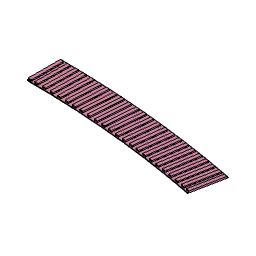
0_15m_Joch_Gebogen_Schablone (Autodesk Fusion 360 design; units mm, degrees)
Autodesk Fusion 360 part; units mm, degrees
sketch "Skizze4" plane through (0, 0, 0) normal (0, 0, 1) x (1, 0, 0)
  line L0 (0, 0) -> (0, -1665.39) construction
  circle A0 centre (0, -1665.39) radius 1665.39 construction
  line L1 (9.1953, 13.0775) -> (9.1001, -0.0222)
  line L2 (9.1001, -0.0222) -> (15.0999, -0.0658)
  line L3 (15.0999, -0.0658) -> (15.1951, 13.0339)
  line L4 (15.1951, 13.0339) -> (9.1953, 13.0775)
  line L5 (-3, 13.1) -> (3, 13.1)
  line L6 (3, 13.1) -> (3, 0)
  line L7 (3, 0) -> (-3, 0)
  line L8 (-3, 0) -> (-3, 13.1)
  line L9 (12.1952, 13.0557) -> (12.1, -0.044) construction
  line L10 (23.708, 12.9352) -> (23.4995, -0.1631)
  line L11 (29.4988, -0.2586) -> (29.7072, 12.8398)
  line L12 (26.7076, 12.8875) -> (26.4992, -0.2108) construction
  line L13 (29.7072, 12.8398) -> (23.708, 12.9352)
  line L14 (23.4995, -0.1631) -> (29.4988, -0.2586)
  line L15 (38.219, 12.6675) -> (37.8973, -0.4285)
  line L16 (58.7237, 12.0751) -> (52.7271, 12.2743)
  line L17 (52.2921, -0.8185) -> (58.2888, -1.0177)
  line L18 (52.7271, 12.2743) -> (52.2921, -0.8185)
  line L19 (58.2888, -1.0177) -> (58.7237, 12.0751)
  line L20 (55.7254, 12.1747) -> (55.2905, -0.9181) construction
  line L21 (41.218, 12.5938) -> (40.8964, -0.5022) construction
  line L22 (37.8973, -0.4285) -> (43.8954, -0.5759)
  line L23 (43.8954, -0.5759) -> (44.2171, 12.5202)
  line L24 (44.2171, 12.5202) -> (38.219, 12.6675)
  line L25 (115.808, -4.0287) -> (116.6954, 9.0412)
  line L26 (101.4385, -3.0895) -> (102.2129, 9.9876)
  line L27 (81.7303, 11.1117) -> (81.0691, -1.9716)
  line L28 (102.2129, 9.9876) -> (96.2234, 10.3423)
  line L29 (67.2312, 11.7557) -> (66.6831, -1.3328)
  line L30 (109.8218, -3.6223) -> (115.808, -4.0287)
  line L31 (87.7227, 10.8088) -> (81.7303, 11.1117)
  line L32 (66.6831, -1.3328) -> (72.6779, -1.5839)
  line L33 (70.2286, 11.6302) -> (69.6805, -1.4584) construction
  line L34 (113.7023, 9.2444) -> (112.8149, -3.8255) construction
  line L35 (81.0691, -1.9716) -> (87.0614, -2.2745)
  line L36 (72.6779, -1.5839) -> (73.226, 11.5046)
  line L37 (84.7265, 10.9602) -> (84.0653, -2.1231) construction
  line L38 (99.2181, 10.165) -> (98.4438, -2.9121) construction
  line L39 (96.2234, 10.3423) -> (95.449, -2.7348)
  line L40 (110.7092, 9.4477) -> (109.8218, -3.6223)
  line L41 (95.449, -2.7348) -> (101.4385, -3.0895)
  line L42 (116.6954, 9.0412) -> (110.7092, 9.4477)
  line L43 (73.226, 11.5046) -> (67.2312, 11.7557)
  line L44 (87.0614, -2.2745) -> (87.7227, 10.8088)
  line L45 (197.4125, 1.4531) -> (195.8485, -11.5532)
  line L46 (139.6549, 7.2828) -> (138.5417, -5.7698)
  line L47 (154.1127, 6.0127) -> (152.8866, -7.0298)
  line L48 (214.793, -0.7) -> (213.1166, -13.6923) construction
  line L49 (173.1887, -9.027) -> (174.5275, 4.0044)
  line L50 (171.5432, 4.3111) -> (170.2044, -8.7204) construction
  line L51 (138.5417, -5.7698) -> (144.52, -6.2797)
  line L52 (152.8866, -7.0298) -> (158.8603, -7.5914)
  line L53 (200.391, 1.095) -> (198.8271, -11.9113) construction
  line L54 (145.6332, 6.7729) -> (139.6549, 7.2828)
  line L55 (211.8177, -0.3161) -> (210.1413, -13.3084)
  line L56 (224.4184, -15.1872) -> (230.3622, -16.0064)
  line L57 (232.1508, -3.0291) -> (226.207, -2.2099)
  line L58 (125.1868, 8.4278) -> (124.1864, -4.634)
  line L59 (182.9926, 3.0978) -> (181.5411, -9.9216)
  line L60 (167.2201, -8.4137) -> (173.1887, -9.027)
  line L61 (217.7683, -1.084) -> (211.8177, -0.3161)
  line L62 (210.1413, -13.3084) -> (216.092, -14.0762)
  line L63 (229.1789, -2.6195) -> (227.3903, -15.5968) construction
  line L64 (185.9741, 2.7654) -> (184.5226, -10.254) construction
  line L65 (131.1692, 7.9696) -> (125.1868, 8.4278)
  line L66 (130.1688, -5.0922) -> (131.1692, 7.9696)
  line L67 (201.8056, -12.2695) -> (203.3696, 0.7368)
  line L68 (160.0864, 5.4511) -> (154.1127, 6.0127)
  line L69 (158.8603, -7.5914) -> (160.0864, 5.4511)
  line L70 (230.3622, -16.0064) -> (232.1508, -3.0291)
  line L71 (168.5589, 4.6177) -> (167.2201, -8.4137)
  line L72 (157.0995, 5.7319) -> (155.8734, -7.3106) construction
  line L73 (188.9556, 2.433) -> (182.9926, 3.0978)
  line L74 (142.6441, 7.0278) -> (141.5308, -6.0248) construction
  line L75 (187.5041, -10.5864) -> (188.9556, 2.433)
  line L76 (128.178, 8.1987) -> (127.1776, -4.8631) construction
  line L77 (203.3696, 0.7368) -> (197.4125, 1.4531)
  line L78 (181.5411, -9.9216) -> (187.5041, -10.5864)
  line L79 (174.5275, 4.0044) -> (168.5589, 4.6177)
  line L80 (195.8485, -11.5532) -> (201.8056, -12.2695)
  line L81 (226.207, -2.2099) -> (224.4184, -15.1872)
  line L82 (144.52, -6.2797) -> (145.6332, 6.7729)
  line L83 (216.092, -14.0762) -> (217.7683, -1.084)
  line L84 (124.1864, -4.634) -> (130.1688, -5.0922)
  line L85 (0, 13.1) -> (0, 0) construction
  line L86 (243.5477, -4.6633) -> (241.6469, -17.6247) construction
  line L87 (275.1899, -9.6098) -> (269.2693, -8.6366)
  line L88 (287.2601, -24.9588) -> (281.3482, -23.9345)
  line L89 (286.5405, -11.539) -> (284.3042, -24.4467) construction
  line L90 (269.2693, -8.6366) -> (267.1446, -21.5632)
  line L91 (246.516, -5.0986) -> (240.5795, -4.228)
  line L92 (281.3482, -23.9345) -> (283.5846, -11.0268)
  line L93 (244.6152, -18.06) -> (246.516, -5.0986)
  line L94 (252.9211, -19.3147) -> (258.8499, -20.2366)
  line L95 (289.4965, -12.0511) -> (287.2601, -24.9588)
  line L96 (240.5795, -4.228) -> (238.6787, -17.1894)
  line L97 (273.0652, -22.5363) -> (275.1899, -9.6098)
  line L98 (258.8499, -20.2366) -> (260.8627, -7.2922)
  line L99 (238.6787, -17.1894) -> (244.6152, -18.06)
  line L100 (254.9339, -6.3703) -> (252.9211, -19.3147)
  line L101 (283.5846, -11.0268) -> (289.4965, -12.0511)
  line L102 (260.8627, -7.2922) -> (254.9339, -6.3703)
  line L103 (272.2296, -9.1232) -> (270.1049, -22.0497) construction
  line L104 (257.8983, -6.8312) -> (255.8855, -19.7757) construction
  line L105 (267.1446, -21.5632) -> (273.0652, -22.5363)
  line L106 (315.0971, -16.7413) -> (312.6378, -29.6084) construction
  line L107 (318.0437, -17.3045) -> (312.1504, -16.1781)
  line L108 (321.6701, -31.3578) -> (327.555, -32.5273)
  line L109 (324.2235, -18.5091) -> (321.6701, -31.3578)
  line L110 (315.5845, -30.1716) -> (318.0437, -17.3045)
  line L111 (312.1504, -16.1781) -> (309.6912, -29.0452)
  line L112 (303.7815, -14.6161) -> (297.8786, -13.5407)
  line L113 (297.8786, -13.5407) -> (295.5307, -26.4286)
  line L114 (295.5307, -26.4286) -> (301.4336, -27.504)
  line L115 (300.83, -14.0784) -> (298.4822, -26.9663) construction
  line L116 (327.166, -19.0938) -> (324.6125, -31.9426) construction
  line L117 (301.4336, -27.504) -> (303.7815, -14.6161)
  line L118 (330.1084, -19.6786) -> (324.2235, -18.5091)
  line L119 (327.555, -32.5273) -> (330.1084, -19.6786)
  line L120 (309.6912, -29.0452) -> (315.5845, -30.1716)
  point P0 (12.1, -0.044)
  point P1 (26.4992, -0.2108)
  point P2 (55.2905, -0.9181)
  point P3 (40.8964, -0.5022)
  point P4 (112.8149, -3.8255)
  point P5 (98.4438, -2.9121)
  point P6 (84.0653, -2.1231)
  point P7 (69.6805, -1.4584)
  point P8 (170.2044, -8.7204)
  point P9 (155.8734, -7.3106)
  point P10 (198.8271, -11.9113)
  point P11 (184.5226, -10.254)
  point P12 (213.1166, -13.6923)
  point P13 (227.3903, -15.5968)
  point P14 (141.5308, -6.0248)
  point P15 (127.1776, -4.8631)
  point P16 (255.8855, -19.7757)
  point P17 (241.6469, -17.6247)
  point P18 (284.3042, -24.4467)
  point P19 (270.1049, -22.0497)
  point P20 (312.6378, -29.6084)
  point P21 (324.6125, -31.9426)
  point P22 (298.4822, -26.9663)
  dimension "d197" = 1665.39
  dimension "d198" = 6
  dimension "d199" = 13.1
  dimension "d200" = 6
  dimension "d201" = 13.1
  dimension "d202" = 6
  dimension "d203" = 13.1
  dimension "d204" = 6
  dimension "d205" = 13.1
  dimension "d206" = 6
  dimension "d207" = 13.1
  dimension "d208" = 6
  dimension "d209" = 13.1
  dimension "d210" = 6
  dimension "d211" = 13.1
  dimension "d212" = 6
  dimension "d213" = 13.1
  dimension "d214" = 6
  dimension "d215" = 13.1
  dimension "d216" = 6
  dimension "d217" = 13.1
  dimension "d218" = 6
  dimension "d219" = 13.1
  dimension "d220" = 6
  dimension "d221" = 13.1
  dimension "d222" = 6
  dimension "d223" = 13.1
  dimension "d224" = 6
  dimension "d225" = 13.1
  dimension "d226" = 6
  dimension "d227" = 13.1
  dimension "d228" = 6
  dimension "d229" = 13.1
  dimension "d230" = 6
  dimension "d231" = 13.1
  dimension "d232" = 12.1
  dimension "d233" = 14.4
  dimension "d234" = 14.4
  dimension "d235" = 14.4
  dimension "d236" = 14.4
  dimension "d237" = 14.4
  dimension "d238" = 14.4
  dimension "d239" = 14.4
  dimension "d240" = 6
  dimension "d241" = 13.1
  dimension "d242" = 6
  dimension "d243" = 13.1
  dimension "d244" = 6
  dimension "d245" = 13.1
  dimension "d246" = 6
  dimension "d247" = 13.1
  dimension "d248" = 6
  dimension "d249" = 13.1
  dimension "d250" = 6
  dimension "d251" = 13.1
  dimension "d252" = 6
  dimension "d253" = 13.1
  dimension "d254" = 14.4
  dimension "d255" = 14.4
  dimension "d256" = 14.4
  dimension "d257" = 14.4
  dimension "d258" = 14.4
  dimension "d259" = 14.4
  dimension "d260" = 14.4
  dimension "d261" = 14.4
  dimension "d262" = 14.4
  dimension "d263" = 14.4
  dimension "d264" = 14.4
  dimension "d265" = 14.4
  dimension "d266" = 14.4
  dimension "d267" = 14.4
  dimension "d268" = 12.2
  dimension "d269" = 11.2
  constraint coincident L0.start L85.end
  constraint vertical L0
  constraint coincident L0.end A0.centre
  constraint coincident L0.start A0
  constraint perpendicular L1 L2
  constraint parallel L1 L3
  constraint parallel L2 L4
  constraint midpoint L2 P0
  constraint horizontal L5
  constraint vertical L6
  constraint horizontal L7
  constraint vertical L8
  constraint midpoint L0.start L7
  constraint midpoint L4 L9.start
  constraint coincident P0 L9.end
  constraint perpendicular L10 L14
  constraint parallel L10 L11
  constraint parallel L13 L14
  constraint midpoint P1 L14
  constraint midpoint L12.start L13
  constraint coincident P1 L12.end
  constraint perpendicular L15 L22
  constraint parallel L15 L23
  constraint parallel L22 L24
  constraint midpoint P3 L22
  constraint midpoint L21.start L24
  constraint coincident P3 L21.end
  constraint perpendicular L17 L18
  constraint parallel L18 L19
  constraint parallel L16 L17
  constraint midpoint P2 L17
  constraint midpoint L20.start L16
  constraint coincident P2 L20.end
  constraint perpendicular L29 L32
  constraint parallel L29 L36
  constraint parallel L32 L43
  constraint midpoint P7 L32
  constraint midpoint L33.start L43
  constraint coincident P7 L33.end
  constraint perpendicular L27 L35
  constraint parallel L27 L44
  constraint parallel L31 L35
  constraint midpoint P6 L35
  constraint midpoint L37.start L31
  constraint coincident P6 L37.end
  constraint perpendicular L39 L41
  constraint parallel L26 L39
  constraint parallel L28 L41
  constraint midpoint P5 L41
  constraint midpoint L38.start L28
  constraint coincident P5 L38.end
  constraint perpendicular L30 L40
  constraint parallel L25 L40
  constraint parallel L30 L42
  constraint midpoint P4 L30
  constraint midpoint L34.start L42
  constraint coincident P4 L34.end
  constraint perpendicular L58 L84
  constraint parallel L58 L66
  constraint parallel L65 L84
  constraint midpoint P15 L84
  constraint midpoint L76.start L65
  constraint coincident P15 L76.end
  constraint perpendicular L46 L51
  constraint parallel L46 L82
  constraint parallel L51 L54
  constraint midpoint P14 L51
  constraint midpoint L74.start L54
  constraint coincident P14 L74.end
  constraint perpendicular L47 L52
  constraint parallel L47 L69
  constraint parallel L52 L68
  constraint midpoint P9 L52
  constraint midpoint L72.start L68
  constraint coincident P9 L72.end
  constraint perpendicular L60 L71
  constraint parallel L49 L71
  constraint parallel L60 L79
  constraint midpoint P8 L60
  constraint midpoint L50.start L79
  constraint coincident P8 L50.end
  constraint perpendicular L59 L78
  constraint parallel L59 L75
  constraint parallel L73 L78
  constraint midpoint P11 L78
  constraint midpoint L64.start L73
  constraint coincident P11 L64.end
  constraint perpendicular L45 L80
  constraint parallel L45 L67
  constraint parallel L77 L80
  constraint midpoint P10 L80
  constraint midpoint L53.start L77
  constraint coincident P10 L53.end
  constraint perpendicular L55 L62
  constraint parallel L55 L83
  constraint parallel L61 L62
  constraint midpoint P12 L62
  constraint midpoint L48.start L61
  constraint coincident P12 L48.end
  constraint perpendicular L56 L81
  constraint parallel L70 L81
  constraint parallel L56 L57
  constraint midpoint P13 L56
  constraint midpoint L63.start L57
  constraint coincident P13 L63.end
  constraint midpoint L5 L85.start
  constraint coincident A0 P0
  constraint coincident A0 P1
  constraint coincident A0 P3
  constraint coincident A0 P2
  constraint coincident A0 P7
  constraint coincident A0 P6
  constraint coincident A0 P5
  constraint coincident A0 P4
  constraint tangent A0 L2
  constraint tangent A0 L14
  constraint tangent A0 L22
  constraint tangent A0 L17
  constraint tangent A0 L32
  constraint tangent A0 L35
  constraint tangent A0 L41
  constraint tangent A0 L30
  constraint coincident A0 P15
  constraint coincident A0 P14
  constraint coincident A0 P9
  constraint coincident A0 P8
  constraint perpendicular L96 L99
  constraint parallel L93 L96
  constraint parallel L91 L99
  constraint midpoint P17 L99
  constraint midpoint L86.start L91
  constraint coincident P17 L86.end
  constraint perpendicular L94 L100
  constraint parallel L98 L100
  constraint parallel L94 L102
  constraint midpoint P16 L94
  constraint midpoint L104.start L102
  constraint coincident P16 L104.end
  constraint perpendicular L90 L105
  constraint parallel L90 L97
  constraint parallel L87 L105
  constraint midpoint P19 L105
  constraint midpoint L103.start L87
  constraint coincident P19 L103.end
  constraint perpendicular L88 L95
  constraint parallel L92 L95
  constraint parallel L88 L101
  constraint midpoint P18 L88
  constraint midpoint L89.start L101
  constraint coincident P18 L89.end
  constraint perpendicular L113 L114
  constraint parallel L113 L117
  constraint parallel L112 L114
  constraint midpoint P22 L114
  constraint midpoint L115.start L112
  constraint coincident P22 L115.end
  constraint perpendicular L111 L120
  constraint parallel L110 L111
  constraint parallel L107 L120
  constraint midpoint P20 L120
  constraint midpoint L106.start L107
  constraint coincident P20 L106.end
  constraint perpendicular L108 L109
  constraint parallel L109 L119
  constraint parallel L108 L118
  constraint midpoint P21 L108
  constraint midpoint L116.start L118
  constraint coincident P21 L116.end
  constraint coincident A0 P11
  constraint coincident A0 P10
  constraint coincident A0 P12
  constraint coincident A0 P13
  constraint tangent A0 L84
  constraint tangent A0 L51
  constraint tangent A0 L52
  constraint tangent A0 L60
  constraint tangent A0 L78
  constraint tangent A0 L80
  constraint tangent A0 L62
  constraint tangent A0 L56
  constraint coincident A0 P17
  constraint coincident A0 P16
  constraint coincident A0 P19
  constraint coincident A0 P18
  constraint coincident A0 P22
  constraint coincident A0 P20
  constraint coincident A0 P21
  constraint tangent A0 L99
  constraint tangent A0 L94
  constraint tangent A0 L105
  constraint tangent A0 L88
  constraint tangent A0 L114
  constraint tangent A0 L120
  constraint tangent A0 L108
  measures "d197" distance of L0.start L0.end
  measures "d198" distance of L1 L3
  measures "d199" distance of L2 L4
  measures "d200" distance of L6 L8
  measures "d201" distance of L5 L7
  measures "d202" distance of L10 L11
  measures "d203" distance of L13 L14
  measures "d204" distance of L15 L23
  measures "d205" distance of L22 L24
  measures "d206" distance of L18 L19
  measures "d207" distance of L16 L17
  measures "d208" distance of L29 L36
  measures "d209" distance of L32 L43
  measures "d210" distance of L27 L44
  measures "d211" distance of L31 L35
  measures "d212" distance of L26 L39
  measures "d213" distance of L28 L41
  measures "d214" distance of L25 L40
  measures "d215" distance of L30 L42
  measures "d216" distance of L58 L66
  measures "d217" distance of L65 L84
  measures "d218" distance of L46 L82
  measures "d219" distance of L51 L54
  measures "d220" distance of L47 L69
  measures "d221" distance of L52 L68
  measures "d222" distance of L49 L71
  measures "d223" distance of L60 L79
  measures "d224" distance of L59 L75
  measures "d225" distance of L73 L78
  measures "d226" distance of L45 L67
  measures "d227" distance of L77 L80
  measures "d228" distance of L55 L83
  measures "d229" distance of L61 L62
  measures "d230" distance of L70 L81
  measures "d231" distance of L56 L57
  measures "d232" distance of P0 L85
  measures "d233" distance of L9 P1
  measures "d234" distance of L12 P3
  measures "d235" distance of P2 L21
  measures "d236" distance of L20 P7
  measures "d237" distance of P6 L33
  measures "d238" distance of P5 L37
  measures "d239" distance of P4 L38
  measures "d240" distance of L93 L96
  measures "d241" distance of L91 L99
  measures "d242" distance of L98 L100
  measures "d243" distance of L94 L102
  measures "d244" distance of L90 L97
  measures "d245" distance of L87 L105
  measures "d246" distance of L92 L95
  measures "d247" distance of L88 L101
  measures "d248" distance of L113 L117
  measures "d249" distance of L112 L114
  measures "d250" distance of L110 L111
  measures "d251" distance of L107 L120
  measures "d252" distance of L109 L119
  measures "d253" distance of L108 L118
  measures "d254" distance of L34 P15
  measures "d255" distance of P14 L76
  measures "d256" distance of P9 L74
  measures "d257" distance of P8 L72
  measures "d258" distance of P11 L50
  measures "d259" distance of P10 L64
  measures "d260" distance of P12 L53
  measures "d261" distance of P13 L48
  measures "d262" distance of L63 P17
  measures "d263" distance of P16 L86
  measures "d264" distance of P19 L104
  measures "d265" distance of P18 L103
  measures "d266" distance of L89 P22
  measures "d267" distance of P20 L115
  measures "d268" distance of P21 L106
extrude "Extrusion1" add sketch "Skizze4" along normal blind 3 makes body 1 at (27.5685, 4.1394, 0) makes body 2 at (83.287, 2.2885, 0) makes body 3 at (140.9055, -1.5889, 0) makes body 4 at (198.3555, -7.4565, 0) makes body 5 at (258.2155, -11.2997, 0) makes body 6 at (312.4754, -25.1316, 0) makes body 7 at (298.281, -22.4911, 0) makes body 8 at (243.2699, -13.4493, 0) makes body 9 at (184.0126, -5.8034, 0) makes body 10 at (126.514, -0.4328, 0) makes body 11 at (68.8641, 2.9463, 0) makes body 12 at (13.1317, 4.3153, 0) makes body 13 at (40.0039, 3.8877, 0) makes body 14 at (97.7036, 1.506, 0) makes body 15 at (155.2865, -2.8695, 0) makes body 16 at (212.6836, -9.2336, 0) makes body 17 at (269.8264, -17.5787, 0) makes body 18 at (327.2956, -23.5717, 0) makes body 19 at (286.7804, -16.0123, 0) makes body 20 at (228.9771, -11.4076, 0) makes body 21 at (169.6559, -4.2743, 0) makes body 22 at (112.4088, 4.9555, 0) makes body 23 at (54.436, 3.4794, 0) makes body 24 at (-1, 4.3667, 0)
move_face "Flächen versetzen1" offset 45.1 24 faces at (297.4984, -26.7871, 1) (240.6575, -17.4796, 1) (183.5288, -10.1432, 1) (126.1805, -4.7867, 1) (83.0665, -2.0726, 1) (25.4993, -0.1949, 1) (254.8974, -19.622, 1) (313.6201, -29.7961, 2) (197.8342, -11.792, 1) (140.5344, -5.9398, 1) (68.6814, -1.4165, 1) (11.1, -0.0367, 1) (39.8967, -0.4777, 1) (97.4455, -2.853, 1) (156.869, -7.4042, 2) (212.1249, -13.5644, 1) (271.0917, -22.2119, 2) (325.5934, -32.1375, 2) (285.2895, -24.6174, 1) (226.3996, -15.4603, 1) (169.2096, -8.6182, 1) (111.8172, -3.7577, 1) (56.2899, -0.9513, 2) (1, 0, 1) on bodies 1 2 3 4 5 6 7 8 9 10 11 12 13 14 15 16 17 18 19 20 21 22 23 24
sketch "Skizze5" plane through (0, 0, 0) normal (0, 0, 1) x (1, 0, 0)
  line L0 (-3, 13.1) -> (-3, -45.1)
  line L1 (318.7642, -76.7623) -> (330.1084, -19.6786)
  line L2 (-3, 13.1) -> (-3, 15.1)
  line L3 (-3, -45.1) -> (-3, -47.1)
  line L4 (330.1084, -19.6786) -> (330.4983, -17.7169)
  line L5 (318.7642, -76.7623) -> (318.3744, -78.7239)
  arc A0 (330.4983, -17.7169) -> (-3, 15.1) centre (-3, -1695.8771) ccw
  arc A1 (318.3744, -78.7239) -> (-3, -47.1) centre (-3, -1695.8771) ccw
  line L6 (-3, 15.1) -> (-30, 15.1)
  line L7 (-3, -47.1) -> (-34, -47.1)
  dimension "d273" = 2
  dimension "d274" = 2
  dimension "d275" = 2
  dimension "d276" = 2
  constraint coincident L0.start L2.start
  constraint coincident L0.end L3.start
  constraint coincident L1.end L4.start
  constraint coincident L1.start L5.start
  constraint parallel L0 L2
  constraint parallel L0 L3
  constraint parallel L1 L5
  constraint parallel L1 L4
  constraint perpendicular L2 L6
  constraint tangent A0 L6
  constraint perpendicular L3 L7
  constraint tangent A1 L7
  measures "d273" distance of L0.start L2.end
  measures "d274" distance of L0.end L3.end
  measures "d275" distance of L1.end L4.end
  measures "d276" distance of L1.start L5.end
extrude "Extrusion2" add sketch "Skizze5" along normal blind 1 separate body makes body 25
combine "Kombinieren1" operation cut target body 25 tool bodies 18 6 7 19 17 5 8 20 16 4 9 21 15 3 10 22 14 2 11 23 13 1 12 24 keep tools
equation "Schwellen_Länge = 58 mm + 0.2 mm"
equation "Schwellen_Breite = 5.8 mm + 0.2 mm"
equation "Bogen_Radius = 1649.39 mm"
equation "Spurweite = 32 mm"
equation "d197 = Bogen_Radius + ( Spurweite / 2 )"
equation "d198 = Schwellen_Breite"
equation "d199 = ( Schwellen_Länge / 2 ) - ( Spurweite / 2 )"
equation "d200 = Schwellen_Breite"
equation "d201 = ( Schwellen_Länge / 2 ) - ( Spurweite / 2 )"
equation "d202 = Schwellen_Breite"
equation "d203 = ( Schwellen_Länge / 2 ) - ( Spurweite / 2 )"
equation "d204 = Schwellen_Breite"
equation "d205 = ( Schwellen_Länge / 2 ) - ( Spurweite / 2 )"
equation "d206 = Schwellen_Breite"
equation "d207 = ( Schwellen_Länge / 2 ) - ( Spurweite / 2 )"
equation "d208 = Schwellen_Breite"
equation "d209 = ( Schwellen_Länge / 2 ) - ( Spurweite / 2 )"
equation "d210 = Schwellen_Breite"
equation "d211 = ( Schwellen_Länge / 2 ) - ( Spurweite / 2 )"
equation "d212 = Schwellen_Breite"
equation "d213 = ( Schwellen_Länge / 2 ) - ( Spurweite / 2 )"
equation "d214 = Schwellen_Breite"
equation "d215 = ( Schwellen_Länge / 2 ) - ( Spurweite / 2 )"
equation "d216 = Schwellen_Breite"
equation "d217 = ( Schwellen_Länge / 2 ) - ( Spurweite / 2 )"
equation "d218 = Schwellen_Breite"
equation "d219 = ( Schwellen_Länge / 2 ) - ( Spurweite / 2 )"
equation "d220 = Schwellen_Breite"
equation "d221 = ( Schwellen_Länge / 2 ) - ( Spurweite / 2 )"
equation "d222 = Schwellen_Breite"
equation "d223 = ( Schwellen_Länge / 2 ) - ( Spurweite / 2 )"
equation "d224 = Schwellen_Breite"
equation "d225 = ( Schwellen_Länge / 2 ) - ( Spurweite / 2 )"
equation "d226 = Schwellen_Breite"
equation "d227 = ( Schwellen_Länge / 2 ) - ( Spurweite / 2 )"
equation "d228 = Schwellen_Breite"
equation "d229 = ( Schwellen_Länge / 2 ) - ( Spurweite / 2 )"
equation "d230 = Schwellen_Breite"
equation "d231 = ( Schwellen_Länge / 2 ) - ( Spurweite / 2 )"
equation "d232 = Schwellen_Abstand_Anfang"
equation "d233 = Schwellen_Abstand_Mitte"
equation "d234 = Schwellen_Abstand_Mitte"
equation "d235 = Schwellen_Abstand_Mitte"
equation "d236 = Schwellen_Abstand_Mitte"
equation "d237 = Schwellen_Abstand_Mitte"
equation "d238 = Schwellen_Abstand_Mitte"
equation "d239 = Schwellen_Abstand_Mitte"
equation "d240 = Schwellen_Breite"
equation "d241 = ( Schwellen_Länge / 2 ) - ( Spurweite / 2 )"
equation "d242 = Schwellen_Breite"
equation "d243 = ( Schwellen_Länge / 2 ) - ( Spurweite / 2 )"
equation "d244 = Schwellen_Breite"
equation "d245 = ( Schwellen_Länge / 2 ) - ( Spurweite / 2 )"
equation "d246 = Schwellen_Breite"
equation "d247 = ( Schwellen_Länge / 2 ) - ( Spurweite / 2 )"
equation "d248 = Schwellen_Breite"
equation "d249 = ( Schwellen_Länge / 2 ) - ( Spurweite / 2 )"
equation "d250 = Schwellen_Breite"
equation "d251 = ( Schwellen_Länge / 2 ) - ( Spurweite / 2 )"
equation "d252 = Schwellen_Breite"
equation "d253 = ( Schwellen_Länge / 2 ) - ( Spurweite / 2 )"
equation "d254 = Schwellen_Abstand_Mitte"
equation "d255 = Schwellen_Abstand_Mitte"
equation "d256 = Schwellen_Abstand_Mitte"
equation "d257 = Schwellen_Abstand_Mitte"
equation "d258 = Schwellen_Abstand_Mitte"
equation "d259 = Schwellen_Abstand_Mitte"
equation "d260 = Schwellen_Abstand_Mitte"
equation "d261 = Schwellen_Abstand_Mitte"
equation "d262 = Schwellen_Abstand_Mitte"
equation "d263 = Schwellen_Abstand_Mitte"
equation "d264 = Schwellen_Abstand_Mitte"
equation "d265 = Schwellen_Abstand_Mitte"
equation "d266 = Schwellen_Abstand_Mitte"
equation "d267 = Schwellen_Abstand_Mitte"
equation "d268 = Schwellen_Abstand_Ende"
equation "d272 = ( Schwellen_Länge / 2 ) + ( Spurweite / 2 )"
equation "d274 = d273"
equation "d275 = d273"
equation "d276 = d273"
equation "Schwellen_Abstand_Anfang = 12.1 mm"
equation "Schwellen_Abstand_Mitte = 14.4 mm"
equation "Schwellen_Abstand_Ende = 12.2 mm"
